Autodesk Inventor part; units mm, degrees
(part 2 of 2)
sketch "Sketch6 outline for Extrusion6" plane through (0, 0, 0) normal (0, 0, 1) x (1, 0, 0)
  line L0 (375.515187, 0) -> (375.315187, 0)
  line L1 (375.315187, 0) -> (375.315187, -6)
  line L2 (375.315187, -6) -> (376.565186, -6)
  line L3 (376.565186, -6) -> (376.565186, -8)
  line L4 (376.565186, -8) -> (375.315187, -8)
  line L5 (375.315187, -8) -> (375.315187, -10.649999)
  line L6 (375.315187, -10.649999) -> (372.315196, -10.649999)
  line L7 (372.315196, -10.649999) -> (372.315196, -8)
  line L8 (372.315196, -8) -> (371.065197, -8)
  line L9 (371.065197, -8) -> (371.065197, -6)
  line L10 (371.065197, -6) -> (372.315196, -6)
  line L11 (372.315196, -6) -> (372.315196, 0)
  line L12 (372.315196, 0) -> (372.115196, 0)
  line L13 (372.115196, 0) -> (372.115196, -5.8)
  line L14 (372.115196, -5.8) -> (370.865197, -5.8)
  line L15 (370.865197, -5.8) -> (370.865197, -8.2)
  line L16 (370.865197, -8.2) -> (372.115196, -8.2)
  line L17 (372.115196, -8.2) -> (372.115196, -10.849999)
  line L18 (372.115196, -10.849999) -> (375.515187, -10.849999)
  line L19 (375.515187, -10.849999) -> (375.515187, -8.2)
  line L20 (375.515187, -8.2) -> (376.765186, -8.2)
  line L21 (376.765186, -8.2) -> (376.765186, -5.8)
  line L22 (376.765186, -5.8) -> (375.515187, -5.8)
  line L23 (375.515187, -5.8) -> (375.515187, 0)
  line L24 (75.397436, -394.000844) -> (74.147437, -394.000851)
  line L25 (75.397424, -392.000843) -> (75.397436, -394.000844)
  line L26 (74.147426, -392.000851) -> (75.397424, -392.000843)
  line L27 (74.14741, -389.350851) -> (74.147426, -392.000851)
  line L28 (71.147419, -389.350868) -> (74.14741, -389.350851)
  line L29 (71.147434, -392.000868) -> (71.147419, -389.350868)
  line L30 (69.897436, -392.000875) -> (71.147434, -392.000868)
  line L31 (69.897447, -394.000875) -> (69.897436, -392.000875)
  line L32 (71.147446, -394.000868) -> (69.897447, -394.000875)
  line L33 (71.14748, -400.000868) -> (71.147446, -394.000868)
  line L34 (70.94748, -400.000869) -> (71.14748, -400.000868)
  line L35 (70.947479, -399.800869) -> (70.94748, -400.000869)
  line L36 (70.947447, -394.200869) -> (70.947479, -399.800869)
  line L37 (69.697448, -394.200876) -> (70.947447, -394.200869)
  line L38 (69.697434, -391.800876) -> (69.697448, -394.200876)
  line L39 (70.947433, -391.800869) -> (69.697434, -391.800876)
  line L40 (70.947418, -389.150869) -> (70.947433, -391.800869)
  line L41 (74.347409, -389.15085) -> (70.947418, -389.150869)
  line L42 (74.347424, -391.800849) -> (74.347409, -389.15085)
  line L43 (75.597423, -391.800842) -> (74.347424, -391.800849)
  line L44 (75.597437, -394.200843) -> (75.597423, -391.800842)
  line L45 (74.347438, -394.20085) -> (75.597437, -394.200843)
  line L46 (74.34747, -399.80085) -> (74.347438, -394.20085)
  line L47 (74.347471, -400.00085) -> (74.34747, -399.80085)
  line L48 (74.147471, -400.000851) -> (74.347471, -400.00085)
  line L49 (74.147437, -394.000851) -> (74.147471, -400.000851)
  line L50 (376.766273, -391.799135) -> (375.516274, -391.799142)
  line L51 (375.516274, -391.799142) -> (375.516259, -389.149143)
  line L52 (375.516259, -389.149143) -> (372.116268, -389.149162)
  line L53 (372.116268, -389.149162) -> (372.116283, -391.799161)
  line L54 (372.116283, -391.799161) -> (370.866284, -391.799169)
  line L55 (370.866284, -391.799169) -> (370.866298, -394.199169)
  line L56 (370.866298, -394.199169) -> (372.116297, -394.199162)
  line L57 (372.116297, -394.199162) -> (372.116331, -400.199162)
  line L58 (372.116331, -400.199162) -> (375.516322, -400.199143)
  line L59 (375.516322, -400.199143) -> (375.516288, -394.199143)
  line L60 (375.516288, -394.199143) -> (376.766287, -394.199135)
  line L61 (376.766287, -394.199135) -> (376.766273, -391.799135)
  line L62 (376.566286, -393.999137) -> (375.316287, -393.999144)
  line L63 (375.316287, -393.999144) -> (375.316321, -399.999144)
  line L64 (375.316321, -399.999144) -> (372.31633, -399.999161)
  line L65 (372.31633, -399.999161) -> (372.316296, -393.999161)
  line L66 (372.316296, -393.999161) -> (371.066297, -393.999168)
  line L67 (371.066297, -393.999168) -> (371.066286, -391.999167)
  line L68 (371.066286, -391.999167) -> (372.316284, -391.99916)
  line L69 (372.316284, -391.99916) -> (372.316269, -389.349161)
  line L70 (372.316269, -389.349161) -> (375.316261, -389.349144)
  line L71 (375.316261, -389.349144) -> (375.316276, -391.999143)
  line L72 (375.316276, -391.999143) -> (376.566274, -391.999136)
  line L73 (376.566274, -391.999136) -> (376.566286, -393.999137)
  line L74 (75.595235, -5.800843) -> (74.345236, -5.80085)
  line L75 (75.595249, -8.200843) -> (75.595235, -5.800843)
  line L76 (74.345236, -5.80085) -> (74.345202, 0.19915)
  line L77 (74.34525, -8.20085) -> (75.595249, -8.200843)
  line L78 (74.345202, 0.19915) -> (70.945211, 0.199131)
  line L79 (74.345265, -10.850849) -> (74.34525, -8.20085)
  line L80 (70.945211, 0.199131) -> (70.945245, -5.800869)
  line L81 (70.945274, -10.850869) -> (74.345265, -10.850849)
  line L82 (70.945245, -5.800869) -> (69.695246, -5.800876)
  line L83 (70.945259, -8.200869) -> (70.945274, -10.850869)
  line L84 (69.695246, -5.800876) -> (69.69526, -8.200876)
  line L85 (69.69526, -8.200876) -> (70.945259, -8.200869)
  line L86 (69.895247, -6.000875) -> (71.145246, -6.000868)
  line L87 (69.895259, -8.000875) -> (69.895247, -6.000875)
  line L88 (71.145258, -8.000868) -> (69.895259, -8.000875)
  line L89 (71.145273, -10.650867) -> (71.145258, -8.000868)
  line L90 (74.145264, -10.65085) -> (71.145273, -10.650867)
  line L91 (74.145249, -8.000851) -> (74.145264, -10.65085)
  line L92 (75.395248, -8.000844) -> (74.145249, -8.000851)
  line L93 (75.395236, -6.000844) -> (75.395248, -8.000844)
  line L94 (74.145237, -6.000851) -> (75.395236, -6.000844)
  line L95 (74.145203, -0.000851) -> (74.145237, -6.000851)
  line L96 (71.145212, -0.000868) -> (74.145203, -0.000851)
  line L97 (71.145246, -6.000868) -> (71.145212, -0.000868)
extrude "Extrusion6" cut sketch "Sketch6 outline for Extrusion6" against normal blind 25.4
body "Solid1"
